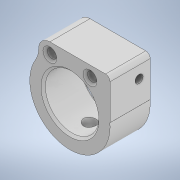
# Autodesk Inventor part: hold pen - slider pen
Saved by Autodesk Inventor 2020 (Build 240168000, 168)
## iProperties
Created: 2026-07-08
Part Number: hold pen - slider pen
Material: Generic
Document SubType Name: Modeling
Designer: drago
Density: 1 g/cm^3
Appearance: Default
Author: drago
Autodesk Inventor part; units mm, degrees
ref_plane "YZ Plane" through (0, 0, 0) normal (1, 0, 0) x (0, 1, 0)
ref_plane "XZ Plane" through (0, 0, 0) normal (0, 1, 0) x (-1, 0, 0)
sketch "Sketch1" plane through (0, 0, 0) normal (0, 0, 1) x (1, 0, 0)
  circle A0 centre (9, 0) radius 1
  circle A1 centre (0, 0) radius 1
  line L0 (0, 2.5) -> (9, 2.5)
  arc A2 (0, 2.5) -> (-2.5, 0) centre (0, 0) ccw
  arc A3 (11.5, 0) -> (9, 2.5) centre (9, 0) ccw
  arc A4 (-3.2143, -2.5754) -> (-2.5, 0) centre (-7.5, 0) ccw
  arc A5 (11.5, 0) -> (12.2143, -2.5754) centre (16.5, 0) ccw
  arc A6 (-3.2143, -2.5754) -> (-4.1458, -4.7111) centre (4.5, -7.2111) ccw
  line L1 (-8.5, -4.7111) -> (-4.1458, -4.7111)
  line L2 (13.1458, -4.7111) -> (17.5, -4.7111)
  line L3 (17.5, -9.7111) -> (13.1458, -9.7111)
  line L4 (-4.1458, -9.7111) -> (-8.5, -9.7111)
  line L5 (17.5, -7.9611) -> (10.4529, -7.9611)
  line L6 (-1.4529, -7.9611) -> (-8.5, -7.9611)
  line L7 (-8.5, -6.4611) -> (-1.4529, -6.4611)
  line L8 (10.4529, -6.4611) -> (17.5, -6.4611)
  arc A7 (-4.1458, -9.7111) -> (13.1458, -9.7111) centre (4.5, -7.2111) ccw
  arc A8 (13.1458, -4.7111) -> (12.2143, -2.5754) centre (4.5, -7.2111) ccw
  arc A9 (-1.4529, -7.9611) -> (10.4529, -7.9611) centre (4.5, -7.2111) ccw
  arc A10 (10.4529, -6.4611) -> (-1.4529, -6.4611) centre (4.5, -7.2111) ccw
  line L9 (17.5, -4.7111) -> (17.5, -6.4611)
  line L10 (17.5, -7.9611) -> (17.5, -9.7111)
  line L11 (-8.5, -9.7111) -> (-8.5, -7.9611)
  line L12 (-8.5, -6.4611) -> (-8.5, -4.7111)
  constraints: 26 end point, 18 point on circle, 12 parallel, 11 centre point, 4 horizontal, 4 perpendicular, 3 coincident, 3 tangent, 1 equal radius
extrude "Extrusion1" add sketch "Sketch1" along normal blind 5
sketch "Sketch2" plane through (13.1458, -9.7111, 0) normal (0, -1, 0) x (1, 0, 0)
  line L0 (4.3542, 0) -> (4.3542, 5) projected
  line L1 (0, 0) -> (0, 5) projected
  circle A0 centre (2.1771, 2.5) radius 0.9
  circle A1 centre (-19.4687, 2.5) radius 0.9
  point P0 (-13.1458, 0)
  dimension "d13" = 1.8
  constraints: 2 centre point
  measures "d13" diameter of A0
extrude "Extrusion2" cut sketch "Sketch2" against normal blind 5
fillet "Fillet1" radius 0.8 8 edges at (17.5, -4.7111, 2.5) (17.5, -9.7111, 2.5) (-8.5, -4.7111, 2.5) (-8.5, -9.7111, 2.5) (17.5, -6.4611, 2.5) (17.5, -7.9611, 2.5) (-8.5, -7.9611, 2.5) (-8.5, -6.4611, 2.5)
fillet "Fillet2" radius 0.8 4 edges at (-1.4529, -6.4611, 2.5) (10.4529, -6.4611, 2.5) (10.4529, -7.9611, 2.5) (-1.4529, -7.9611, 2.5)
sketch "Sketch3" plane through (0, 0, 5) normal (0, 0, 1) x (1, 0, 0)
  arc A0 (11.5, 0) -> (9, 2.5) centre (9, 0) ccw projected
  line L0 (14.4229, -6.4611) -> (14.4229, -4.7111) projected
  line L1 (9, 2.5) -> (14.4229, 2.5)
  line L2 (14.4229, 2.5) -> (14.4229, -4.7111)
  line L3 (14.4229, -4.7111) -> (9, -4.7111)
  line L4 (9, -4.7111) -> (9, 2.5)
  arc A1 (13.1458, -4.7111) -> (12.2143, -2.5754) centre (4.5, -7.2111) ccw projected
  arc A2 (11.5, 0) -> (12.2143, -2.5754) centre (16.5, 0) ccw projected
  point P0 (0, 0)
  constraints: 8 end point, 2 parallel, 1 horizontal, 1 perpendicular, 1 point on line
extrude "Extrusion3" add sketch "Sketch3" against normal blind 5 contours A0 L1 L2 L3 A1 A2
sketch "Sketch4" plane through (14.4229, -4.7111, 5) normal (1, 0, 0) x (0, 0, -1)
  line L0 (0, 0) -> (0, 7.2111) projected
  line L1 (2.5, 0) -> (0, 0) projected
  line L2 (5, 0) -> (2.5, 0) projected
  line L3 (5, 7.2111) -> (5, 0) projected
  line L4 (0, 7.2111) -> (5, 7.2111) projected
  point P0 (5, 4.7111)
extrude "Extrusion4" cut sketch "Sketch4" against normal blind 0.923
sketch "Sketch5" plane through (13.4999, -4.7111, 5) normal (1, 0, 0) x (0, 0, -1)
  line L0 (0, 3.5) -> (5, 3.5) projected
  circle A0 centre (2.5, 3.5) radius 0.9
  point P0 (5, 4.7111)
  dimension "d25" = 1.8
  constraints: 1 centre point, 1 midpoint
  measures "d25" diameter of A0
extrude "Extrusion5" cut sketch "Sketch5" against normal blind 2.5
fillet "Fillet3" radius 1 1 edges at (13.4999, 2.5, 2.5)
sketch "Sketch6" plane through (0, 0, 5) normal (0, 0, 1) x (1, 0, 0)
  arc A0 (-1.342, -8.5787) -> (10.342, -8.5787) centre (4.5, -7.2111) ccw projected
  circle A1 centre (4.5, -7.2111) radius 6
  circle A2 centre (4.5, -7.2111) radius 9
  line L0 (13.4999, -4.7111) -> (13.4999, 1.5) projected
  line L1 (13.4999, -4.7111) -> (17.88, -4.7111)
  line L2 (17.88, -4.7111) -> (17.88, -10.4948)
  line L3 (17.88, -10.4948) -> (13.4999, -10.4948)
  line L4 (13.4999, -10.4948) -> (13.4999, -4.7111)
  line L5 (-4.1458, -4.7111) -> (-7.7, -4.7111) projected
  line L6 (-4.1458, -4.7111) -> (-9.7441, -4.7111)
  line L7 (-9.7441, -4.7111) -> (-9.7441, -9.7121)
  line L8 (-9.7441, -9.7121) -> (-4.1458, -9.7121)
  line L9 (-4.1458, -9.7121) -> (-4.1458, -4.7111)
  line L10 (13.4999, -10.4948) -> (12.8796, -10.4948)
  point P0 (0, 0)
  point P1 (-4.1458, -9.7111)
  point P2 (13.4999, -7.1696)
  constraints: 18 end point, 4 parallel, 3 horizontal, 2 centre point, 2 coincident, 2 perpendicular, 1 point on circle
extrude "Extrusion6" cut sketch "Sketch6" against normal blind 10 contours L4 L10 A2 | L4 L1 L2 L3 | A2 L8 L7 L6 L5
sketch "Sketch7" plane through (0, 0, 5) normal (0, 0, 1) x (1, 0, 0)
  arc A0 (-1.342, -8.5787) -> (10.342, -8.5787) centre (4.5, -7.2111) ccw projected
  circle A1 centre (4.5, -7.2111) radius 6
  circle A2 centre (4.5, -7.2111) radius 9
  line L0 (-4.4687, -6.4611) -> (-2.121, -6.4611) projected
  arc A3 (-2.121, -6.4611) -> (-1.342, -5.8435) centre (-2.121, -5.6611) ccw projected
  line L1 (-2.121, -7.9611) -> (-4.4687, -7.9611) projected
  arc A4 (-1.342, -8.5787) -> (-2.121, -7.9611) centre (-2.121, -8.7611) ccw projected
  line L2 (11.121, -6.4611) -> (13.4999, -6.4611) projected
  arc A5 (10.342, -5.8435) -> (11.121, -6.4611) centre (11.121, -5.6611) ccw projected
  arc A6 (11.121, -7.9611) -> (10.342, -8.5787) centre (11.121, -8.7611) ccw projected
  line L3 (13.4687, -7.9611) -> (11.121, -7.9611) projected
  point P0 (0, 0)
  point P1 (13.4687, -6.4611)
  point P2 (10.342, -8.5787)
  point P3 (-1.342, -8.5787)
  constraints: 2 centre point, 2 coincident
extrude "Extrusion7" add sketch "Sketch7" against normal up to surface (5 mm away) contours A4 L1 A2 L0 A3 A1 | A1 A5 L2 A2 L3 A6
sketch "Sketch8" plane through (0, 0, 5) normal (0, 0, 1) x (1, 0, 0)
  circle A0 centre (4.5, -7.2111) radius 6 projected
  circle A1 centre (0, 0) radius 1 projected
  circle A2 centre (9, 0) radius 1 projected
  arc A3 (-3.2143, -2.5754) -> (13.4687, -6.4611) centre (4.5, -7.2111) ccw projected
  line L0 (13.4687, -6.4611) -> (13.4999, -6.4611) projected
  line L1 (13.4999, -6.4611) -> (13.4999, 1.5) projected
  arc A4 (13.4999, 1.5) -> (12.4999, 2.5) centre (12.4999, 1.5) ccw projected
  line L2 (12.4999, 2.5) -> (0, 2.5) projected
  arc A5 (0, 2.5) -> (-2.5, 0) centre (0, 0) ccw projected
  arc A6 (-3.2143, -2.5754) -> (-2.5, 0) centre (-7.5, 0) ccw projected
extrude "Extrusion8" add sketch "Sketch8" along normal blind 4
ref_plane "Work Plane1" through (0, -22.25, 0) normal (0, 1, 0) x (1, 0, 0)
sketch "Sketch9" plane through (0, -22.25, 0) normal (0, 1, 0) x (1, 0, 0)
  line L0 (-4.5, -9) -> (13.5, -9) projected
  line L1 (13.5, 0) -> (13.5, -9) projected
  circle A0 centre (4.5, -4.5) radius 1.4
  point P0 (0, 0)
  point P1 (-3.2143, -9)
  point P2 (13.4687, -9)
  dimension "d36" = 2.8
  constraints: 1 centre point
  measures "d36" diameter of A0
extrude "Extrusion9" cut sketch "Sketch9" along normal blind 10
chamfer "Chamfer2" distance 0.5 angle 45 2 edges at (4.5, -13.2111, 0) (-1.5, -7.2111, 9)
sketch "Sketch10" plane through (0, 0, 0) normal (0, 0, -1) x (-1, 0, 0)
  circle A0 centre (0, 0) radius 1.05
  circle A1 centre (-9, 0) radius 1 projected
  circle A2 centre (-9, 0) radius 1.05
  dimension "d42" = 2.1
  dimension "d43" = 2.1
  constraints: 2 centre point, 2 coincident
  measures "d42" diameter of A0
  measures "d43" diameter of A2
extrude "Extrusion10" cut sketch "Sketch10" against normal blind 10
chamfer "Chamfer3" distance 0.5 angle 45 4 edges at (1.05, 0, 0) (10.05, 0, 0) (1.05, 0, 9) (10.05, 0, 9)
body "Solid1"
